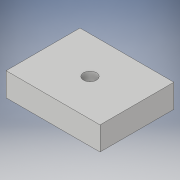
# Autodesk Inventor part: SINGLE HOLE CONNECTOR
Saved by Autodesk Inventor 2019 (Build 230136000, 136)
## iProperties
Created: 2019-05-04
Part Number: SINGLE HOLE CONNECTOR
Material: Generic
Document SubType Name: Modeling
Designer: User
Density: 1 g/cm^3
Appearance: Default
Author: User
Autodesk Inventor part; units mm, degrees
ref_plane "YZ Plane" through (0, 0, 0) normal (1, 0, 0) x (0, 1, 0)
ref_plane "XZ Plane" through (0, 0, 0) normal (0, 1, 0) x (-1, 0, 0)
ref_plane "XY Plane" through (0, 0, 0) normal (0, 0, 1) x (1, 0, 0)
sketch "Sketch1" plane through (0, 0, 0) normal (0, 1, 0) x (-1, 0, 0)
  line L0 (0, 0) -> (25.4, 0)
  line L1 (25.4, 0) -> (25.4, -19.9898)
  line L2 (25.4, -19.9898) -> (0, -19.9898)
  line L3 (0, -19.9898) -> (0, 0)
  dimension "d0" = 25.4
  dimension "d1" = 19.9898
  constraints: 8 end point, 2 parallel, 1 horizontal, 1 perpendicular
  measures "d0" distance of L1.end L2.end
  measures "d1" distance of L0.end L1.end
extrude "Extrusion1" add sketch "Sketch1" along normal blind 6.35
sketch "Sketch2" plane through (0, 6.35, 0) normal (0, 1, 0) x (1, 0, 0)
  line L0 (-25.4, 0) -> (0, 0) projected
  line L1 (0, 0) -> (0, 19.9898) projected
  line L2 (0, 19.9898) -> (-25.4, 19.9898) projected
  line L3 (-25.4, 19.9898) -> (-25.4, 0) projected
  point P0 (-12.7, 9.9949)
  dimension "d4" = 19.9898
  dimension "d5" = 25.4
  dimension "d6" = 12.7
  dimension "d7" = 9.9949
  measures "d4" distance of L2.end L0.start
  measures "d5" distance of L1.end L2.end
  measures "d6" distance from line of L3 point (-12.7, 9.995)
  measures "d7" distance from line of L2 point (-12.7, 9.995)
hole "Hole1" at (-12.7, 6.35, -9.9949) direction (0, -1, 0) diameter 3.5052 end through all
equation "\"d6\" = 0.5 * d5"
equation "\"d7\" = 0.5 * d4"
body "Solid1"
